Autodesk Inventor part; units mm, degrees
(part 2 of 2)
sketch "Sketch17" plane through (0, 3.175, 0) normal (0, 1, 0) x (1, 0, 0)
  line L0 (-193.2102, -16.6805) -> (-155.0467, -16.6805) construction
  line L1 (-155.0467, -16.6805) -> (-155.0467, -30.1673) construction
  line L2 (-155.0467, -30.1673) -> (-193.2102, -30.1673) construction
  line L3 (-193.2102, -30.1673) -> (-193.2102, -16.6805) construction
  line L4 (-200.8302, -13.1267) -> (-200.8302, -33.721) projected
  line L5 (-200.8302, -23.4239) -> (-144.5457, -23.4239) construction
  line L6 (-190.191, -26.439) -> (-190.191, -20.4746)
  line L7 (-190.191, -20.4746) -> (-189.2219, -20.4088)
  spline S0 degree 2 poles (-189.2219, -20.4088) (-188.498, -20.4088) (-188.0733, -20.8574) knots 0 0 0 1 1 1
  spline S1 degree 2 poles (-188.0733, -20.8574) (-187.6545, -21.3121) (-187.6545, -22.0061) knots 0 0 0 1 1 1
  spline S2 degree 2 poles (-187.6545, -22.0061) (-187.6545, -22.8795) (-188.4143, -23.2623) knots 0 0 0 1 1 1
  spline S3 degree 2 poles (-188.4143, -23.2623) (-187.1939, -23.5375) (-187.1939, -24.8477) knots 0 0 0 1 1 1
  spline S4 degree 2 poles (-187.1939, -24.8477) (-187.1939, -25.5117) (-187.5947, -26.0082) knots 0 0 0 1 1 1
  spline S5 degree 2 poles (-187.5947, -26.0082) (-188.0015, -26.5048) (-188.9108, -26.5048) knots 0 0 0 1 1 1
  spline S6 degree 2 poles (-188.9108, -26.5048) (-189.2398, -26.5048) (-189.6346, -26.4689) knots 0 0 0 1 1 1
  spline S7 degree 2 poles (-189.6346, -26.4689) (-189.9816, -26.439) (-190.191, -26.439) knots 0 0 0 1 1 1
  line L8 (-189.1561, -23.5615) -> (-189.7244, -23.5615)
  line L9 (-189.7244, -23.5615) -> (-189.7244, -24.5785)
  spline S8 degree 2 poles (-189.7244, -24.5785) (-189.7244, -25.6433) (-189.4911, -25.9305) knots 0 0 0 1 1 1
  spline S9 degree 2 poles (-189.4911, -25.9305) (-189.2937, -26.08) (-188.8988, -26.08) knots 0 0 0 1 1 1
  spline S10 degree 2 poles (-188.8988, -26.08) (-188.2348, -26.08) (-187.9476, -25.6972) knots 0 0 0 1 1 1
  spline S11 degree 2 poles (-187.9476, -25.6972) (-187.6784, -25.3143) (-187.6784, -24.7998) knots 0 0 0 1 1 1
  spline S12 degree 2 poles (-187.6784, -24.7998) (-187.6784, -24.387) (-187.8519, -24.0939) knots 0 0 0 1 1 1
  spline S13 degree 2 poles (-187.8519, -24.0939) (-188.0374, -23.7948) (-188.3066, -23.6751) knots 0 0 0 1 1 1
  spline S14 degree 2 poles (-188.3066, -23.6751) (-188.5937, -23.5615) (-189.1561, -23.5615) knots 0 0 0 1 1 1
  line L10 (-190.6038, -20.4746) -> (-190.6038, -26.439)
  spline S15 degree 2 poles (-190.6038, -26.439) (-191.1003, -26.4569) (-191.7943, -26.5048) knots 0 0 0 1 1 1
  line L11 (-191.7943, -26.5048) -> (-191.7943, -26.4031)
  spline S16 degree 2 poles (-191.7943, -26.4031) (-191.0704, -26.2057) (-191.0704, -24.8716) knots 0 0 0 1 1 1
  line L12 (-191.0704, -24.8716) -> (-191.0704, -21.9223)
  spline S17 degree 2 poles (-191.0704, -21.9223) (-191.0704, -20.7498) (-191.7943, -20.5105) knots 0 0 0 1 1 1
  line L13 (-191.7943, -20.5105) -> (-191.7943, -20.4088)
  spline S18 degree 2 poles (-191.7943, -20.4088) (-191.208, -20.4626) (-190.6038, -20.4746) knots 0 0 0 1 1 1
  line L14 (-189.7244, -22.024) -> (-189.7244, -23.1606)
  line L15 (-189.7244, -23.1606) -> (-189.2877, -23.1606)
  spline S19 degree 2 poles (-189.2877, -23.1606) (-188.7433, -23.1606) (-188.4501, -22.8675) knots 0 0 0 1 1 1
  spline S20 degree 2 poles (-188.4501, -22.8675) (-188.151, -22.5744) (-188.151, -22.018) knots 0 0 0 1 1 1
  spline S21 degree 2 poles (-188.151, -22.018) (-188.151, -21.4437) (-188.4741, -21.1446) knots 0 0 0 1 1 1
  spline S22 degree 2 poles (-188.4741, -21.1446) (-188.7911, -20.8515) (-189.2338, -20.8515) knots 0 0 0 1 1 1
  spline S23 degree 2 poles (-189.2338, -20.8515) (-189.4731, -20.8515) (-189.6227, -20.9711) knots 0 0 0 1 1 1
  spline S24 degree 2 poles (-189.6227, -20.9711) (-189.7244, -21.2762) (-189.7244, -22.024) knots 0 0 0 1 1 1
  spline S25 degree 2 poles (-187.2956, -26.2774) (-186.7751, -25.733) (-186.7751, -24.8776) knots 0 0 0 1 1 1
  spline S26 degree 2 poles (-186.7751, -24.8776) (-186.7751, -23.9623) (-187.3195, -23.3999) knots 0 0 0 1 1 1
  spline S27 degree 2 poles (-187.3195, -23.3999) (-186.2427, -23.7888) (-186.2427, -24.8297) knots 0 0 0 1 1 1
  spline S28 degree 2 poles (-186.2427, -24.8297) (-186.2427, -25.3442) (-186.5418, -25.745) knots 0 0 0 1 1 1
  spline S29 degree 2 poles (-186.5418, -25.745) (-186.8409, -26.1458) (-187.2956, -26.2774) knots 0 0 0 1 1 1
  spline S30 degree 2 poles (-187.5767, -23.0829) (-187.2297, -22.6282) (-187.2297, -22.0061) knots 0 0 0 1 1 1
  spline S31 degree 2 poles (-187.2297, -22.0061) (-187.2297, -21.5155) (-187.4212, -21.1207) knots 0 0 0 1 1 1
  spline S32 degree 2 poles (-187.4212, -21.1207) (-187.6246, -20.7198) (-187.8818, -20.5823) knots 0 0 0 1 1 1
  spline S33 degree 2 poles (-187.8818, -20.5823) (-187.3195, -20.7019) (-187.0204, -21.0668) knots 0 0 0 1 1 1
  spline S34 degree 2 poles (-187.0204, -21.0668) (-186.7212, -21.4317) (-186.7212, -21.8804) knots 0 0 0 1 1 1
  spline S35 degree 2 poles (-186.7212, -21.8804) (-186.7212, -22.2753) (-186.9725, -22.6282) knots 0 0 0 1 1 1
  spline S36 degree 2 poles (-186.9725, -22.6282) (-187.2178, -22.9692) (-187.5767, -23.0829) knots 0 0 0 1 1 1
  spline S37 degree 2 poles (-179.6741, -23.4239) (-179.6741, -24.4708) (-179.9911, -25.1887) knots 0 0 0 1 1 1
  spline S38 degree 2 poles (-179.9911, -25.1887) (-180.3022, -25.9006) (-180.8705, -26.2415) knots 0 0 0 1 1 1
  spline S39 degree 2 poles (-180.8705, -26.2415) (-181.4209, -26.5885) (-182.1627, -26.5885) knots 0 0 0 1 1 1
  spline S40 degree 2 poles (-182.1627, -26.5885) (-183.3412, -26.5885) (-183.9873, -25.745) knots 0 0 0 1 1 1
  spline S41 degree 2 poles (-183.9873, -25.745) (-184.6334, -24.9015) (-184.6334, -23.4239) knots 0 0 0 1 1 1
  spline S42 degree 2 poles (-184.6334, -23.4239) (-184.6334, -21.8864) (-183.9754, -21.0668) knots 0 0 0 1 1 1
  spline S43 degree 2 poles (-183.9754, -21.0668) (-183.3173, -20.2592) (-182.1747, -20.2592) knots 0 0 0 1 1 1
  spline S44 degree 2 poles (-182.1747, -20.2592) (-181.0201, -20.2592) (-180.3441, -21.0668) knots 0 0 0 1 1 1
  spline S45 degree 2 poles (-180.3441, -21.0668) (-179.6741, -21.8685) (-179.6741, -23.4239) knots 0 0 0 1 1 1
  spline S46 degree 2 poles (-180.2065, -23.4298) (-180.2065, -20.7198) (-182.1747, -20.7198) knots 0 0 0 1 1 1
  spline S47 degree 2 poles (-182.1747, -20.7198) (-184.107, -20.7198) (-184.107, -23.5016) knots 0 0 0 1 1 1
  spline S48 degree 2 poles (-184.107, -23.5016) (-184.107, -26.1159) (-182.1567, -26.1159) knots 0 0 0 1 1 1
  spline S49 degree 2 poles (-182.1567, -26.1159) (-180.2065, -26.1159) (-180.2065, -23.4298) knots 0 0 0 1 1 1
  spline S50 degree 2 poles (-184.442, -21.001) (-185.0641, -21.9642) (-185.0641, -23.4657) knots 0 0 0 1 1 1
  spline S51 degree 2 poles (-185.0641, -23.4657) (-185.0641, -24.8237) (-184.4719, -25.8228) knots 0 0 0 1 1 1
  spline S52 degree 2 poles (-184.4719, -25.8228) (-185.6145, -25.069) (-185.6145, -23.4119) knots 0 0 0 1 1 1
  spline S53 degree 2 poles (-185.6145, -23.4119) (-185.6145, -21.7069) (-184.442, -21.001) knots 0 0 0 1 1 1
  spline S54 degree 2 poles (-179.8775, -25.8527) (-179.2613, -25.0152) (-179.2613, -23.3281) knots 0 0 0 1 1 1
  spline S55 degree 2 poles (-179.2613, -23.3281) (-179.2613, -21.8385) (-179.8715, -21.007) knots 0 0 0 1 1 1
  spline S56 degree 2 poles (-179.8715, -21.007) (-178.7109, -21.7069) (-178.7109, -23.394) knots 0 0 0 1 1 1
  spline S57 degree 2 poles (-178.7109, -23.394) (-178.7109, -25.057) (-179.8775, -25.8527) knots 0 0 0 1 1 1
  line L16 (-174.4814, -26.439) -> (-174.625, -26.439)
  line L17 (-174.625, -26.439) -> (-174.625, -20.4746)
  line L18 (-174.625, -20.4746) -> (-172.591, -20.4746)
  spline S58 degree 2 poles (-172.591, -20.4746) (-172.0286, -20.4746) (-171.4902, -20.4088) knots 0 0 0 1 1 1
  spline S59 degree 2 poles (-171.4902, -20.4088) (-171.4902, -20.5164) (-171.5022, -20.7976) knots 0 0 0 1 1 1
  spline S60 degree 2 poles (-171.5022, -20.7976) (-171.5201, -21.0549) (-171.5201, -21.4497) knots 0 0 0 1 1 1
  spline S61 degree 2 poles (-171.5201, -21.4497) (-171.5201, -21.695) (-171.55, -21.9522) knots 0 0 0 1 1 1
  line L19 (-171.55, -21.9522) -> (-171.6876, -21.9522)
  spline S62 degree 2 poles (-171.6876, -21.9522) (-171.6996, -21.4856) (-171.915, -21.1805) knots 0 0 0 1 1 1
  spline S63 degree 2 poles (-171.915, -21.1805) (-172.1423, -20.8694) (-172.8721, -20.8694) knots 0 0 0 1 1 1
  line L20 (-172.8721, -20.8694) -> (-174.1583, -20.8694)
  line L21 (-174.1583, -20.8694) -> (-174.1583, -24.9194)
  spline S64 degree 2 poles (-174.1583, -24.9194) (-174.1583, -25.6194) (-173.9609, -25.9664) knots 0 0 0 1 1 1
  spline S65 degree 2 poles (-173.9609, -25.9664) (-173.7635, -26.3193) (-173.3507, -26.4031) knots 0 0 0 1 1 1
  line L22 (-173.3507, -26.4031) -> (-173.3507, -26.5048)
  spline S66 degree 2 poles (-173.3507, -26.5048) (-174.3498, -26.439) (-174.4814, -26.439) knots 0 0 0 1 1 1
  line L23 (-176.9102, -20.4746) -> (-175.0437, -20.4746)
  line L24 (-175.0437, -20.4746) -> (-175.0437, -26.439)
  line L25 (-175.0437, -26.439) -> (-175.2172, -26.439)
  spline S67 degree 2 poles (-175.2172, -26.439) (-175.5821, -26.439) (-176.312, -26.5048) knots 0 0 0 1 1 1
  line L26 (-176.312, -26.5048) -> (-176.312, -26.4031)
  spline S68 degree 2 poles (-176.312, -26.4031) (-175.8454, -26.2834) (-175.6659, -25.9245) knots 0 0 0 1 1 1
  spline S69 degree 2 poles (-175.6659, -25.9245) (-175.4984, -25.5655) (-175.4984, -24.734) knots 0 0 0 1 1 1
  line L27 (-175.4984, -24.734) -> (-175.4984, -20.8694)
  line L28 (-175.4984, -20.8694) -> (-176.9401, -20.8694)
  spline S70 degree 2 poles (-176.9401, -20.8694) (-177.4905, -20.8694) (-177.7178, -21.0967) knots 0 0 0 1 1 1
  spline S71 degree 2 poles (-177.7178, -21.0967) (-177.9452, -21.3241) (-178.0947, -21.9522) knots 0 0 0 1 1 1
  line L29 (-178.0947, -21.9522) -> (-178.2263, -21.9522)
  spline S72 degree 2 poles (-178.2263, -21.9522) (-178.2323, -21.8744) (-178.2323, -21.7907) knots 0 0 0 1 1 1
  spline S73 degree 2 poles (-178.2323, -21.7907) (-178.2323, -21.677) (-178.2084, -21.5035) knots 0 0 0 1 1 1
  spline S74 degree 2 poles (-178.2084, -21.5035) (-178.1426, -20.8993) (-178.1426, -20.4088) knots 0 0 0 1 1 1
  spline S75 degree 2 poles (-178.1426, -20.4088) (-177.8435, -20.4447) (-177.3948, -20.4566) knots 0 0 0 1 1 1
  line L30 (-177.3948, -20.4566) -> (-176.9102, -20.4746)
  line L31 (-167.3564, -26.439) -> (-167.5, -26.439)
  line L32 (-167.5, -26.439) -> (-167.5, -20.4746)
  line L33 (-167.5, -20.4746) -> (-165.466, -20.4746)
  spline S76 degree 2 poles (-165.466, -20.4746) (-164.9037, -20.4746) (-164.3653, -20.4088) knots 0 0 0 1 1 1
  spline S77 degree 2 poles (-164.3653, -20.4088) (-164.3653, -20.5164) (-164.3772, -20.7976) knots 0 0 0 1 1 1
  spline S78 degree 2 poles (-164.3772, -20.7976) (-164.3952, -21.0549) (-164.3952, -21.4497) knots 0 0 0 1 1 1
  spline S79 degree 2 poles (-164.3952, -21.4497) (-164.3952, -21.695) (-164.4251, -21.9522) knots 0 0 0 1 1 1
  line L34 (-164.4251, -21.9522) -> (-164.5627, -21.9522)
  spline S80 degree 2 poles (-164.5627, -21.9522) (-164.5746, -21.4856) (-164.79, -21.1805) knots 0 0 0 1 1 1
  spline S81 degree 2 poles (-164.79, -21.1805) (-165.0173, -20.8694) (-165.7472, -20.8694) knots 0 0 0 1 1 1
  line L35 (-165.7472, -20.8694) -> (-167.0334, -20.8694)
  line L36 (-167.0334, -20.8694) -> (-167.0334, -24.9194)
  spline S82 degree 2 poles (-167.0334, -24.9194) (-167.0334, -25.6194) (-166.836, -25.9664) knots 0 0 0 1 1 1
  spline S83 degree 2 poles (-166.836, -25.9664) (-166.6385, -26.3193) (-166.2258, -26.4031) knots 0 0 0 1 1 1
  line L37 (-166.2258, -26.4031) -> (-166.2258, -26.5048)
  spline S84 degree 2 poles (-166.2258, -26.5048) (-167.2248, -26.439) (-167.3564, -26.439) knots 0 0 0 1 1 1
  line L38 (-169.7853, -20.4746) -> (-167.9188, -20.4746)
  line L39 (-167.9188, -20.4746) -> (-167.9188, -26.439)
  line L40 (-167.9188, -26.439) -> (-168.0923, -26.439)
  spline S85 degree 2 poles (-168.0923, -26.439) (-168.4572, -26.439) (-169.187, -26.5048) knots 0 0 0 1 1 1
  line L41 (-169.187, -26.5048) -> (-169.187, -26.4031)
  spline S86 degree 2 poles (-169.187, -26.4031) (-168.7204, -26.2834) (-168.5409, -25.9245) knots 0 0 0 1 1 1
  spline S87 degree 2 poles (-168.5409, -25.9245) (-168.3734, -25.5655) (-168.3734, -24.734) knots 0 0 0 1 1 1
  line L42 (-168.3734, -24.734) -> (-168.3734, -20.8694)
  line L43 (-168.3734, -20.8694) -> (-169.8152, -20.8694)
  spline S88 degree 2 poles (-169.8152, -20.8694) (-170.3655, -20.8694) (-170.5929, -21.0967) knots 0 0 0 1 1 1
  spline S89 degree 2 poles (-170.5929, -21.0967) (-170.8202, -21.3241) (-170.9698, -21.9522) knots 0 0 0 1 1 1
  line L44 (-170.9698, -21.9522) -> (-171.1014, -21.9522)
  spline S90 degree 2 poles (-171.1014, -21.9522) (-171.1074, -21.8744) (-171.1074, -21.7907) knots 0 0 0 1 1 1
  spline S91 degree 2 poles (-171.1074, -21.7907) (-171.1074, -21.677) (-171.0834, -21.5035) knots 0 0 0 1 1 1
  spline S92 degree 2 poles (-171.0834, -21.5035) (-171.0176, -20.8993) (-171.0176, -20.4088) knots 0 0 0 1 1 1
  spline S93 degree 2 poles (-171.0176, -20.4088) (-170.7185, -20.4447) (-170.2698, -20.4566) knots 0 0 0 1 1 1
  line L45 (-170.2698, -20.4566) -> (-169.7853, -20.4746)
  line L46 (-159.5674, -26.439) -> (-159.5674, -23.4239)
  line L47 (-159.5674, -23.4239) -> (-162.3971, -20.4746)
  line L48 (-162.3971, -20.4746) -> (-162.2355, -20.4746)
  spline S94 degree 2 poles (-162.2355, -20.4746) (-161.5655, -20.4746) (-160.8417, -20.4088) knots 0 0 0 1 1 1
  line L49 (-160.8417, -20.4088) -> (-160.8417, -20.5105)
  spline S95 degree 2 poles (-160.8417, -20.5105) (-161.1767, -20.6062) (-161.1767, -20.8275) knots 0 0 0 1 1 1
  spline S96 degree 2 poles (-161.1767, -20.8275) (-161.1767, -21.1207) (-160.5007, -21.8266) knots 0 0 0 1 1 1
  line L50 (-160.5007, -21.8266) -> (-159.3042, -23.0769)
  line L51 (-159.3042, -23.0769) -> (-158.1855, -21.7727)
  spline S97 degree 2 poles (-158.1855, -21.7727) (-157.8146, -21.336) (-157.8146, -20.9891) knots 0 0 0 1 1 1
  spline S98 degree 2 poles (-157.8146, -20.9891) (-157.8146, -20.6002) (-158.2035, -20.5105) knots 0 0 0 1 1 1
  line L52 (-158.2035, -20.5105) -> (-158.2035, -20.4088)
  spline S99 degree 2 poles (-158.2035, -20.4088) (-158.0659, -20.4088) (-157.5155, -20.4506) knots 0 0 0 1 1 1
  spline S100 degree 2 poles (-157.5155, -20.4506) (-157.2822, -20.4746) (-157.1027, -20.4746) knots 0 0 0 1 1 1
  spline S101 degree 2 poles (-157.1027, -20.4746) (-157.007, -20.4746) (-156.1096, -20.4088) knots 0 0 0 1 1 1
  line L53 (-156.1096, -20.4088) -> (-156.1096, -20.5105)
  spline S102 degree 2 poles (-156.1096, -20.5105) (-156.5344, -20.6361) (-156.7976, -20.8574) knots 0 0 0 1 1 1
  spline S103 degree 2 poles (-156.7976, -20.8574) (-157.0548, -21.0788) (-157.3839, -21.4736) knots 0 0 0 1 1 1
  spline S104 degree 2 poles (-157.3839, -21.4736) (-157.4018, -21.5035) (-157.4616, -21.5753) knots 0 0 0 1 1 1
  line L54 (-157.4616, -21.5753) -> (-159.1068, -23.4957)
  line L55 (-159.1068, -23.4957) -> (-159.1068, -24.9314)
  spline S105 degree 2 poles (-159.1068, -24.9314) (-159.1068, -26.2415) (-158.2932, -26.4031) knots 0 0 0 1 1 1
  line L56 (-158.2932, -26.4031) -> (-158.2932, -26.5048)
  spline S106 degree 2 poles (-158.2932, -26.5048) (-159.3281, -26.439) (-159.364, -26.439) knots 0 0 0 1 1 1
  line L57 (-159.364, -26.439) -> (-159.5674, -26.439)
  line L58 (-162.9355, -20.4746) -> (-160.0041, -23.5854)
  line L59 (-160.0041, -23.5854) -> (-160.0041, -26.439)
  line L60 (-160.0041, -26.439) -> (-160.1357, -26.439)
  spline S107 degree 2 poles (-160.1357, -26.439) (-160.6323, -26.439) (-161.2724, -26.5048) knots 0 0 0 1 1 1
  line L61 (-161.2724, -26.5048) -> (-161.2724, -26.4031)
  spline S108 degree 2 poles (-161.2724, -26.4031) (-160.9015, -26.3193) (-160.6861, -26.0322) knots 0 0 0 1 1 1
  spline S109 degree 2 poles (-160.6861, -26.0322) (-160.4767, -25.751) (-160.4767, -24.9553) knots 0 0 0 1 1 1
  line L62 (-160.4767, -24.9553) -> (-160.4767, -23.717)
  line L63 (-160.4767, -23.717) -> (-162.2774, -21.8146)
  spline S110 degree 2 poles (-162.2774, -21.8146) (-163.3064, -20.7378) (-164.1379, -20.5105) knots 0 0 0 1 1 1
  line L64 (-164.1379, -20.5105) -> (-164.1379, -20.4088)
  spline S111 degree 2 poles (-164.1379, -20.4088) (-163.6653, -20.4746) (-163.1209, -20.4746) knots 0 0 0 1 1 1
  line L65 (-163.1209, -20.4746) -> (-162.9355, -20.4746)
  point P0 (0, 0)
  point P1 (-193.2102, -23.4239)
  dimension "d206" = 7.62
  constraints: 2 end point, 2 midpoint, 1 horizontal, 1 point on line, 2 other
  measures "d206" distance between parallel lines of L4 L3
emboss "Emboss2" sketch "Sketch17" operation add depth 0.2 direction (0, -1, 0)
sketch "Sketch13" plane through (0, 3.175, 0) normal (0, 1, 0) x (1, 0, 0)
  line L0 (-100.2262, -38.2104) -> (-100.2262, -157.352) construction
  line L1 (-100.2262, -157.352) -> (-143.0309, -157.352) construction
  line L2 (-143.0309, -157.352) -> (-143.0309, -38.2104) construction
  line L3 (-143.0309, -38.2104) -> (-100.2262, -38.2104) construction
  line L4 (-144.2491, -33.721) -> (-144.2491, -142.941) projected
  point P0 (0, 0)
  constraints: 1 parallel, 2 other
equation "\"d11\" = d9"
equation "\"d12\" = d10"
equation "\"d53\" = d11"
equation "\"d9\" = 144.1069"
body "Solid1"
